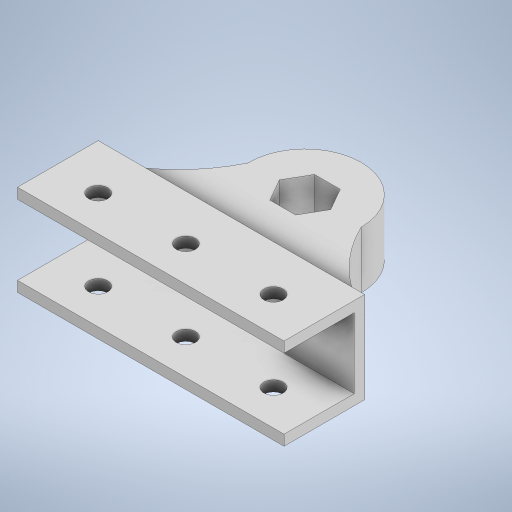
# Autodesk Inventor part: CH-1-02-BearingBracket
Saved by Autodesk Inventor 2023.1 (Build 271208000, 208)
## iProperties
Created: 2023-02-19
Part Number: CH-1-02-BearingBracket
Material: Generic
Document SubType Name: Modeling
Designer: eplym
Density: 1 g/cm^3
Appearance: Default
Author: eplym
Autodesk Inventor part; units mm, degrees
ref_plane "YZ Plane" through (0, 0, 0) normal (1, 0, 0) x (0, 1, 0)
ref_plane "XZ Plane" through (0, 0, 0) normal (0, 1, 0) x (-1, 0, 0)
ref_plane "XY Plane" through (0, 0, 0) normal (0, 0, 1) x (1, 0, 0)
sketch "Sketch1" plane through (0, 0, 0) normal (0, 1, 0) x (-1, 0, 0)
  line L0 (-38, 30) -> (38, 30)
  line L1 (38, 30) -> (38, -30)
  line L2 (38, -30) -> (-38, -30)
  line L3 (-38, -30) -> (-38, 30)
  line L4 (-38, 30) -> (38, -30) construction
  line L5 (38, 30) -> (-38, -30) construction
  point P0 (0, 0)
  dimension "d0" = 60
  dimension "d1" = 76
  constraints: 12 end point, 2 midpoint, 2 parallel, 1 horizontal, 1 perpendicular
  measures "d0" distance of L0.end L1.end
  measures "d1" distance of L1.end L2.end
extrude "Extrusion1" add sketch "Sketch1" along normal blind 26
sketch "Sketch2" plane through (-38, 0, 30) normal (0, 0, 1) x (1, 0, 0)
  line L0 (0, 0) -> (0, 26) projected
  line L1 (76, 0) -> (76, 26) projected
  line L2 (0, 23) -> (76, 23)
  line L3 (76, 23) -> (76, 3)
  line L4 (76, 3) -> (0, 3)
  line L5 (0, 3) -> (0, 23)
  line L6 (0, 26) -> (76, 26) projected
  line L7 (0, 0) -> (76, 0) projected
  point P0 (38, 0)
  point P1 (0, 3)
  dimension "d4" = 3
  dimension "d5" = 3
  constraints: 8 end point, 2 parallel, 2 point on line, 1 horizontal, 1 perpendicular
  measures "d4" distance between parallel lines of L6 L2
  measures "d5" distance between parallel lines of L7 L4
extrude "Extrusion2" cut sketch "Sketch2" against normal blind 20 contours L0 L2 L1 L4
sketch "Sketch3" plane through (0, 26, 0) normal (0, 1, 0) x (1, 0, 0)
  arc A0 (15.9974, 14) -> (-16, 13.7099) centre (-0.0026, 14) ccw
  line L0 (38, 30) -> (-38, 30) projected
  line L1 (-38, 30) -> (-38, -30) projected
  arc A1 (-38, -7) -> (-16, 13.7099) centre (-54.3067, 32.3627) ccw
  line L2 (38, -30) -> (38, 30) projected
  line L3 (38, 30) -> (-38, 30) projected
  line L4 (38, -30) -> (-38, -30) projected
  arc A2 (15.9974, 14) -> (38, -7) centre (54.478, 32.2913) ccw
  line L5 (-38, -10) -> (-38, -30) projected
  line L6 (-38, -7) -> (38, -7)
  line L7 (38, -10) -> (-38, -10) projected
  point P0 (0, 0)
  point P1 (38, -7)
  point P2 (-0.0026, 30)
  dimension "d8" = 32
  dimension "d10" = 3
  constraints: 6 point on circle, 3 centre point, 2 end point, 1 parallel, 1 point on line, 1 tangent
  measures "d8" diameter of A0
  measures "d10" distance between parallel lines of L6 L7
extrude "Extrusion3" cut sketch "Sketch3" against normal through all contours A0 L0 L2 A2 | A0 A1 L1 L0
sketch "Sketch5" plane through (0, 26, 0) normal (0, 1, 0) x (1, 0, 0)
  arc A0 (15.9974, 14) -> (-16, 13.7099) centre (-0.0026, 14) ccw
  line L0 (38, 30) -> (-38, 30)
  line L1 (-38, 30) -> (-38, -30)
  arc A1 (-38, -7) -> (-16, 13.7099) centre (-54.3067, 32.3627) ccw
  line L2 (38, -30) -> (38, 30)
  line L3 (38, 30) -> (-38, 30)
  line L4 (38, -30) -> (-38, -30)
  arc A2 (15.9974, 14) -> (38, -7) centre (54.478, 32.2913) ccw
  line L5 (-38, -10) -> (-38, -30)
  line L6 (-38, -7) -> (38, -7)
  line L7 (38, -10) -> (-38, -10)
  point P0 (0, 0)
  point P1 (0, 0)
  point P2 (38, -7)
  point P3 (-0.0026, 30)
  dimension "d13" = 32
  dimension "d14" = 3
  constraints: 16 end point, 6 point on circle, 3 centre point, 1 parallel, 1 point on line, 1 tangent
  measures "d13" diameter of A0
  measures "d14" distance between parallel lines of L6 L7
sketch "Sketch7" plane through (0, 0, 0) normal (0, -1, 0) x (1, 0, 0)
  arc A0 (-16, -13.7099) -> (15.9974, -14) centre (-0.0026, -14) ccw projected
  arc A1 (-16, -13.7099) -> (15.9974, -14) centre (-0.0026, -14) ccw
  line L0 (38, 30) -> (38, 7) projected
  arc A2 (38, 7) -> (15.9974, -14) centre (54.478, -32.2913) ccw
  arc A3 (-16, -13.7099) -> (-38, 7) centre (-54.3067, -32.3627) ccw projected
  arc A4 (-16, -13.7099) -> (-38, 7) centre (-54.3067, -32.3627) ccw
  line L1 (-38, 10) -> (38, 10) projected
  line L2 (38, 10) -> (-38, 10)
  line L3 (38, 7) -> (38, 10)
  line L4 (-38, 7) -> (-38, 30) projected
  line L5 (-38, 7) -> (-38, 10)
  arc A5 (38, 7) -> (15.9974, -14) centre (54.478, -32.2913) ccw projected
  line L6 (38, 7) -> (-38, 7)
  point P0 (0, 0)
  constraints: 8 end point, 7 point on circle, 3 centre point, 3 collinear, 1 coincident, 1 horizontal
extrude "Extrusion4" cut sketch "Sketch5" against normal blind 4.875 contours A2 L6 A1 A0
extrude "Extrusion5" cut sketch "Sketch7" against normal blind 4.875 contours A3 L6 A2 A0
sketch "Sketch9" plane through (0, 21.125, 0) normal (0, 1, 0) x (1, 0, 0)
  arc A0 (15.9974, 14) -> (-16, 13.7099) centre (-0.0026, 14) ccw projected
  line L0 (3.6635, 20.35) -> (7.3297, 14)
  line L1 (7.3297, 14) -> (3.6635, 7.65)
  line L2 (3.6635, 7.65) -> (-3.6688, 7.65)
  line L3 (-3.6688, 7.65) -> (-7.335, 14)
  line L4 (-7.335, 14) -> (-3.6688, 20.35)
  line L5 (-3.6688, 20.35) -> (3.6635, 20.35)
  point P0 (0, 0)
  dimension "d19" = 12.7
  constraints: 12 end point, 1 coincident, 13 other
  measures "d19" distance between parallel lines of L2 L5
extrude "Extrusion6" cut sketch "Sketch9" against normal through all
sketch "Sketch10" plane through (0, 26, 0) normal (0, 1, 0) x (1, 0, 0)
  circle A0 centre (0, -20) radius 5.8489
  circle A1 centre (25, -20) radius 5.871
  circle A2 centre (-25, -20) radius 5.8765
  line L0 (-38, -7) -> (-38, -30) projected
  line L1 (-38, -30) -> (38, -30) projected
  point P0 (0, 0)
  dimension "d23" = 10
  dimension "d24" = 10
  dimension "d25" = 10
  dimension "d27" = 0
  dimension "d28" = 25
  dimension "d29" = 25
  constraints: 3 centre point
  measures "d23" distance from line of L1 A0.centre
  measures "d24" distance from line of L1 A1.centre
  measures "d25" distance from line of L1 A2.centre
  measures "d27" horizontal distance of A0.centre point (0, 0)
  measures "d28" distance of A0.centre A2.centre
  measures "d29" distance of A0.centre A1.centre
hole "Hole1" at (-25, 26, 20) at (0, 26, 20) at (25, 26, 20) direction (0, -1, 0) diameter 5.5 end through all clearance for "Flat Head Machine Screw" size "M5" standard "Ansi Metric M Profile"
body "Solid1"
